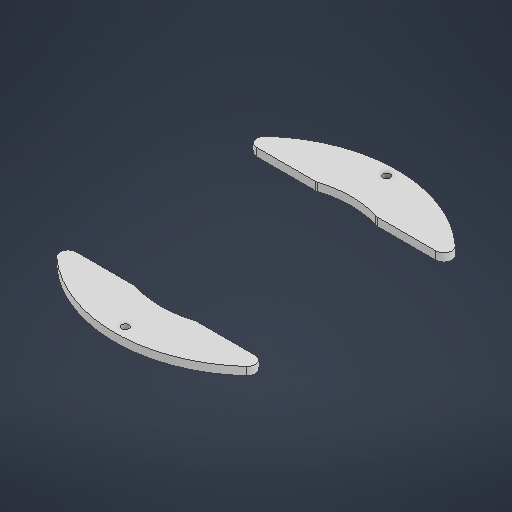
# Autodesk Inventor part: Cylinder Segment Holder Both Cameras
Saved by Autodesk Inventor 2026 (Build 300175000, 175)
## iProperties
Created: 2025-05-08
Part Number: Cylinder Segment Holder Both Cameras
Material: Generic
Document SubType Name: Modeling
Designer: Charl
Density: 1 g/cm^3
Appearance: Default
Author: Charl
Autodesk Inventor part; units mm, degrees
ref_plane "YZ Plane" through (0, 0, 0) normal (1, 0, 0) x (0, 1, 0)
ref_plane "XZ Plane" through (0, 0, 0) normal (0, 1, 0) x (-1, 0, 0)
ref_plane "XY Plane" through (0, 0, 0) normal (0, 0, 1) x (1, 0, 0)
sketch "Sketch1" plane through (0, 0, 0) normal (0, 1, 0) x (-1, 0, 0)
  circle A0 centre (0, 0) radius 59
  circle A1 centre (0, 0) radius 81
  circle A2 centre (0, 0) radius 87.5
  circle A3 centre (0, 81) radius 2.25
  circle A4 centre (0, -81) radius 2.25
  line L0 (90, -56) -> (15, -56)
  line L1 (10, -51) -> (10, 51)
  line L2 (15, 56) -> (90, 56)
  line L3 (90, 56) -> (90, -56)
  line L4 (90, -56) -> (10, 56) construction
  line L5 (10, -56) -> (90, 56) construction
  arc A5 (10, -51) -> (15, -56) centre (15, -51) ccw
  arc A6 (15, 56) -> (10, 51) centre (15, 51) ccw
  line L6 (0, 103.0841) -> (0, -103.0841)
  line L7 (-90, -56) -> (-15, -56)
  line L8 (-10, -51) -> (-10, 51)
  line L9 (-15, 56) -> (-90, 56)
  line L10 (-90, 56) -> (-90, -56)
  arc A7 (-15, -56) -> (-10, -51) centre (-15, -51) ccw
  arc A8 (-10, 51) -> (-15, 56) centre (-15, 51) ccw
  point P0 (50, 0)
  point P1 (90, 0)
  point P2 (10, 0)
  point P3 (56.2614, -45.3902)
  point P4 (56.2614, 63.4399)
  point P5 (76.2614, 44.4685)
  point P6 (76.2614, -26.4188)
  point P7 (63.4942, 65.0248)
  point P8 (63.4942, -46.9752)
  point P9 (67.2328, 56)
  point P10 (-67.2328, 56)
  point P11 (-18.5742, 56)
  point P12 (18.5742, 56)
  point P13 (18.5742, -56)
  point P14 (-18.5742, -56)
  point P15 (-67.2328, -56)
  point P16 (67.2328, -56)
  dimension "d0" = 118
  dimension "d1" = 162
  dimension "d2" = 175
  dimension "d3" = 4.5
  dimension "d4" = 4.5
  dimension "d5" = 112
  dimension "d6" = 80
  dimension "d7" = 10
  dimension "d8" = 5
  dimension "d9" = 0
  dimension "d10" = 0
  dimension "d11" = 56
  constraints: 22 end point, 10 point on circle, 9 centre point, 8 symmetric about line, 5 midpoint, 4 point on line, 4 tangent, 3 coincident, 2 parallel, 1 equal radius, 1 horizontal, 1 perpendicular, 1 vertical, 2 other
  measures "d0" diameter of A0
  measures "d1" diameter of A1
  measures "d2" diameter of A2
  measures "d3" diameter of A3
  measures "d4" diameter of A4
  measures "d5" distance of L4.end L5.start
  measures "d6" distance of L4.end L2.end
  measures "d7" distance of point (0, 0) point (10, 0)
  measures "d8" radius of A5
  measures "d9" distance of point (0, 0) point (0, 0)
  measures "d10" distance of point (0, 0) A0.centre
  measures "d11" distance from line of point (0, 0) L0
extrude "Extrusion1" add sketch "Sketch1" along normal blind 5 contours A0 L6 A3 A1 L2 | L0 A1 A4 L6 A0 | A0 L9 A1 A3 L6 | A1 A3 L6 A2 L2 | L6 A4 A1 L7 A0 | L0 A2 L6 A4 A1 | L9 A2 L6 A3 A1 | A1 A4 L6 A2 L7
fillet "Fillet1" radius 5 8 edges at (-67.2328, 2.5, -56) (-18.5742, 2.5, -56) (-67.2328, 2.5, 56) (-18.5742, 2.5, 56) (18.5742, 2.5, 56) (67.2328, 2.5, 56) (18.5742, 2.5, -56) (67.2328, 2.5, -56)
equation "\"d11\" = 0.5 * d5"
body "Solid1"
